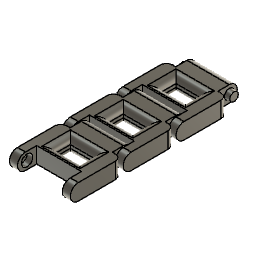
gyakorlati 10 lancszemek (Autodesk Fusion 360 design; units mm, degrees)
Autodesk Fusion 360 part; units mm, degrees
sketch "Sketch1" plane through (0, 0, 0) normal (0, 0, 1) x (1, 0, 0)
  line L0 (0, 0) -> (0, 16)
  line L1 (0, 0) -> (7, 0)
  line L2 (7, 0) -> (7, -6)
  line L3 (7, -6) -> (9.5, -6)
  line L4 (9.5, -6) -> (9.5, 10)
  line L5 (9.5, 10) -> (6.6, 10)
  line L6 (6.6, 10) -> (6.6, 16)
  line L7 (6.6, 16) -> (0, 16)
  dimension "d1" = 16
  dimension "d2" = 7
  dimension "d3" = 2.5
  dimension "d4" = 2.9
  constraint coincident L0.start L1.start
  constraint vertical L0
  constraint perpendicular L0 L1
  constraint perpendicular L1 L2
  constraint perpendicular L2 L3
  constraint perpendicular L3 L4
  constraint perpendicular L4 L5
  constraint perpendicular L5 L6
  constraint perpendicular L0 L7
  measures "d1" distance of L0.start L0.end
  measures "d2" distance of L0.start L1.end
  measures "d3" distance of L2.end L3.end
  measures "d4" distance of L4.end L5.end
extrude "Extrude1" add sketch "Sketch1" along normal blind 5 makes body 1
fillet "Fillet1" radius 2.5 4 edges at (8.25, -6, 5) (8.25, -6, 0) (3.3, 16, 5) (3.3, 16, 0) on bodies 1
sketch "Sketch2" plane through (6.6, 0, 0) normal (1, 0, 0) x (0, 1, 0)
  arc A0 (13.5, 0) -> (13.5, 5) centre (13.5, 2.5) ccw
  line L0 (13.5, 5) -> (10, 5)
  line L1 (10, 5) -> (10, 0)
  line L2 (10, 0) -> (13.5, 0)
  circle A1 centre (13.5, 2.5) radius 1.5
  constraint concentric A0 A1
extrude "Extrude2" add sketch "Sketch2" along normal blind 1.5 draft -7 contours A1 bodies 1
sketch "Sketch3" plane through (7, 0, 0) normal (-1, 0, 0) x (0, -1, 0)
  arc A0 (3.5, 0) -> (3.5, 5) centre (3.5, 2.5) ccw
  line L0 (3.5, 5) -> (0, 5)
  line L1 (0, 5) -> (0, 0)
  line L2 (0, 0) -> (3.5, 0)
  line L3 (0, 2.5) -> (3, 2.5) construction
  circle A1 centre (3, 2.5) radius 1.75
  dimension "d11" = 3
  dimension "d12" = 3.5
  constraint midpoint L1 L3.start
  constraint perpendicular L1 L3
  constraint coincident L3.end A1.centre
  measures "d11" distance of L3.start L3.end
  measures "d12" diameter of A1
extrude "Extrude3" cut sketch "Sketch3" against normal up to surface (1.6 mm away) draft -7 contours A1 bodies 1
sketch "Sketch4" plane through (0, 0, 5) normal (0, 0, 1) x (-1, 0, 0)
  line L0 (-6.6, -13.5) -> (0, -13.5)
  line L1 (0, -13.5) -> (0, 0)
  line L2 (0, 0) -> (-7, 0)
  line L3 (-7, 0) -> (-7, 3.5)
  line L4 (-7, 3.5) -> (-9.5, 3.5)
  line L5 (-9.5, 3.5) -> (-9.5, -10)
  line L6 (-9.5, -10) -> (-6.6, -10)
  line L7 (-6.6, -10) -> (-6.6, -13.5)
  line L8 (0, -2.5) -> (-4, -2.5)
  line L9 (-4, -2.5) -> (-4, -7.5)
  line L10 (-4, -7.5) -> (0, -7.5)
  line L11 (0, -7.5) -> (0, -2.5)
  dimension "d15" = 4
  dimension "d16" = 5
  dimension "d17" = 2.5
  constraint horizontal L8
  constraint vertical L9
  constraint horizontal L10
  constraint vertical L11
  constraint coincident L1 L8.start
  measures "d15" distance of L8.start L8.end
  measures "d16" distance of L8.start L10.end
  measures "d17" distance of L2 L8
extrude "Extrude4" cut sketch "Sketch4" against normal blind 9 contours L1 L8 L9 L10 L11 bodies 1
mirror "Mirror1" about plane through (0, 0, 0) normal (1, 0, 0) of bodies 1 merged
fillet "Fillet2" radius 2 8 edges at (0, 7.5, 5) (-4, 5, 5) (0, 2.5, 5) (4, 5, 5) (0, 2.5, 0) (4, 5, 0) (-4, 5, 0) (0, 7.5, 0) on bodies 1
fillet "Fillet3" radius 2 2 edges at (-9.5, 10, 2.5) (9.5, 10, 2.5) on bodies 1
pattern_linear "R-Pattern1" count 3 spacing 16.5 along (0, -1, 0) of bodies 1 makes body 2 at (-2, -4.333, 0) makes body 3 at (-2, -20.833, 0)
copy_body "CutPasteBodies1" bodies 1 2 3 removing the originals makes body 4 makes body 5 makes body 6 in component "sbu"
component "sbu" placed x (1, 0, 0) y (0, 1, 0) z (0, 0, 1) at (0, 0, 0)
